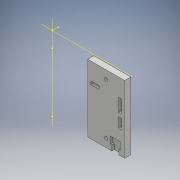
# Autodesk Inventor part: 1구버전
Saved by Autodesk Inventor 2018 (Build 220112000, 112)
## iProperties
Created: 2018-01-17
Part Number: 1구버전
Material: 일반
Document SubType Name: Modeling
Designer: NULL
Density: 1 g/cm^3
Appearance: 기본값
Author: NULL
Autodesk Inventor part; units mm, degrees
ref_plane "작업 평면1" through (0, 10, 0) normal (0, 1, 0) x (1, 0, 0)
sketch "스케치3" plane through (0, 10, 0) normal (0, 1, 0) x (1, 0, 0)
  line L0 (108.4435, 113.2704) -> (97.4435, 113.2704)
  line L1 (97.4435, 113.2704) -> (97.4435, 121.7204)
  line L2 (97.4435, 121.7204) -> (108.4435, 121.7204)
  line L3 (108.4435, 121.7204) -> (108.4435, 113.2704)
  line L4 (117.9435, 121.7204) -> (57.9435, 121.7204)
  line L5 (57.9435, 121.7204) -> (57.9435, 11.7204)
  line L6 (117.9435, 11.7204) -> (117.9435, 121.7204)
  line L7 (57.9435, 11.7204) -> (117.9435, 11.7204)
  line L8 (113.0685, 67.6907) -> (89.4185, 67.6907)
  line L9 (89.4185, 67.6907) -> (89.4185, 84.1907)
  line L10 (89.4185, 84.1907) -> (113.0685, 84.1907)
  line L11 (113.0685, 84.1907) -> (113.0685, 67.6907)
  line L12 (113.0684, 40.1407) -> (108.0685, 40.1407)
  line L13 (108.0685, 67.6907) -> (113.0685, 67.6907)
  line L14 (113.0684, 61.6907) -> (113.0684, 40.1407)
  line L15 (113.0685, 67.6907) -> (108.0685, 67.6907)
  line L16 (108.0685, 67.6907) -> (108.0685, 84.1907)
  line L17 (108.0685, 84.1907) -> (113.0685, 84.1907)
  line L18 (113.0685, 84.1907) -> (113.0685, 67.6907)
  line L19 (76.5185, 39.8907) -> (62.8185, 39.8907)
  line L20 (62.8185, 39.8907) -> (62.8185, 44.8907)
  line L21 (62.8185, 44.8907) -> (76.5185, 44.8907)
  line L22 (76.5185, 44.8907) -> (76.5185, 39.8907)
  line L23 (113.0684, 61.6907) -> (78.3675, 61.6907)
  circle A0 centre (87.9435, 25.2204) radius 2.6
  circle A1 centre (87.9435, 108.2204) radius 2.6
  line L24 (78.3675, 40.1407) -> (113.0684, 40.1407)
  line L25 (78.3675, 40.1407) -> (78.3675, 61.6907)
  line L26 (76.5185, 39.8907) -> (76.5185, 71.6407)
  line L27 (62.8185, 39.8907) -> (62.8185, 71.6407)
  line L28 (76.5185, 71.6407) -> (62.8185, 71.6407)
  line L29 (108.0685, 61.6907) -> (108.0685, 40.1407)
  point P0 (0, 0)
  dimension "d8" = 9.5
  dimension "d46" = 5.2
  dimension "d47" = 5.2
  constraints: 60 end point, 8 parallel, 6 horizontal, 4 perpendicular, 4 point on line, 2 centre point, 1 collinear, 1 vertical
  measures "d8" distance of L4.start L2.end
  measures "d46" diameter of A0
  measures "d47" diameter of A1
extrude "돌출2" add sketch "스케치3" against normal blind 10 contours L3 L4 L6 L7 L5 L1 L0 | L0 L1 L2 L3 | L8 L16 L10 L11 | L8 L9 L10 L16 | L12 L29 L23 L14 | L24 L25 L23 L29 | L19 L20 L21 L22 | L21 L27 L28 L26 | A0 | A1
sketch "스케치4" plane through (0, 10, 0) normal (0, 1, 0) x (1, 0, 0)
  point P0 (0, 0)
sketch "스케치5" plane through (117.9435, 10, -121.7204) normal (0, 0, -1) x (-1, 0, 0)
  point P0 (117.9435, -10)
extrude "돌출5" cut sketch "스케치3" against normal through all contours L0 L1 L2 L3
sketch "스케치6" plane through (0, 0, 0) normal (0, -1, 0) x (1, 0, 0)
  line L0 (57.9435, -121.7204) -> (97.4435, -121.7204) projected
  line L1 (97.4435, -121.7204) -> (57.9435, -121.7204) projected
  line L2 (113.0685, -71.6204) -> (108.0685, -71.6204) projected
  line L3 (113.0685, -80.2704) -> (113.0685, -71.6204) projected
  line L4 (78.3685, -80.2704) -> (113.0685, -80.2704) projected
  line L5 (78.3685, -58.4704) -> (78.3685, -80.2704) projected
  line L6 (113.0685, -58.4704) -> (78.3685, -58.4704) projected
  line L7 (113.0685, -67.1204) -> (113.0685, -58.4704) projected
  line L8 (108.0685, -67.1204) -> (113.0685, -67.1204) projected
  line L9 (108.0685, -71.6204) -> (108.0685, -67.1204) projected
  line L10 (117.9435, -121.7204) -> (108.4435, -121.7204) projected
  line L11 (111.4435, -108.7204) -> (94.443, -108.7204)
  line L12 (111.4435, -108.7204) -> (111.4435, -113.2704)
  line L13 (94.443, -108.7204) -> (94.443, -113.2704)
  line L14 (111.4435, -113.2704) -> (94.443, -113.2704)
  point P0 (0, 0)
  constraints: 8 end point, 2 vertical, 1 perpendicular
sketch "스케치7" plane through (0, 0, 0) normal (0, -1, 0) x (1, 0, 0)
  point P0 (0, 0)
sketch "스케치8" plane through (0, 0, 0) normal (0, -1, 0) x (1, 0, 0)
  point P0 (0, 0)
extrude "돌출6" cut sketch "스케치6" against normal blind 4 contours L12 L14 L13 L11
extrude "돌출7" add sketch "스케치3" against normal blind 6 contours L0 L1 L2 L3
sketch "스케치9" plane through (0, 0, 0) normal (0, -1, 0) x (1, 0, 0)
  line L0 (111.4435, -108.7204) -> (111.4435, -113.2704) projected
  line L1 (111.4435, -108.7204) -> (111.4435, -101.7204)
  line L2 (111.4435, -101.7204) -> (94.443, -101.7204)
  line L3 (94.443, -113.2704) -> (94.443, -108.7204) projected
  line L4 (94.443, -101.7204) -> (94.443, -108.7204)
  line L5 (94.443, -108.7204) -> (111.4435, -108.7204) projected
  line L6 (111.4435, -108.7204) -> (94.443, -108.7204)
  point P0 (0, 0)
  dimension "d25" = 7
  constraints: 8 end point, 2 perpendicular, 1 collinear, 1 vertical
  measures "d25" distance of L0.start L1.end
extrude "돌출8" cut sketch "스케치9" against normal blind 4
sketch "스케치10" plane through (0, 10, 0) normal (0, 1, 0) x (1, 0, 0)
  circle A0 centre (87.9435, 25.2204) radius 3.85
  circle A1 centre (87.9435, 108.2204) radius 3.85
  point P0 (0, 0)
  dimension "d28" = 7.7
  dimension "d29" = 7.7
  constraints: 2 centre point
  measures "d28" diameter of A0
  measures "d29" diameter of A1
ref_plane "작업 평면2" through (0, 10, 0) normal (0, 1, 0) x (1, 0, 0)
sketch "스케치12" plane through (0, 10, 0) normal (0, 1, 0) x (1, 0, 0)
  point P0 (0, 0)
ref_plane "작업 평면3" through (57.9435, 10, -25.2204) normal (0, 0, 1) x (1, 0, 0)
sketch "스케치13" plane through (57.9435, 10, -25.2204) normal (0, 0, 1) x (1, 0, 0)
  line L0 (30, 0) -> (30, -4)
  line L1 (30, 0) -> (33.65, 0)
  line L2 (33.65, 0) -> (30, -4)
  point P0 (-57.9435, -10)
  point P1 (32.25, 0)
  dimension "d35" = 4
  dimension "d36" = 3.65
  constraints: 6 end point, 1 vertical
  measures "d35" distance of L0.start L0.end
  measures "d36" distance of L0.start L1.end
sketch "스케치14" plane through (57.9435, 10, -25.2204) normal (0, 0, 1) x (1, 0, 0)
  point P0 (-57.9435, -10)
revolve "회전2" cut sketch "스케치13" angle 360 about axis through (87.9435, 10, -25.2204) along (0, -1, 0)
ref_plane "작업 평면4" through (57.9435, 10, -66.7204) normal (0, 0, 1) x (1, 0, 0)
mirror "미러1" about plane through (57.9435, 10, -66.7204) normal (0, 0, 1) of "회전2"
sketch "스케치15" plane through (0, 0, 0) normal (0, -1, 0) x (1, 0, 0)
  line L0 (108.6612, -121.7204) -> (97.1612, -121.7204)
  line L1 (97.1612, -121.7204) -> (97.1612, -113.2704)
  line L2 (108.6612, -121.7204) -> (108.6612, -113.2704)
  line L3 (97.1612, -113.2704) -> (108.6612, -113.2704)
  line L4 (97.4435, -113.2704) -> (94.443, -113.2704) projected
  point P0 (0, 0)
  constraints: 8 end point, 2 vertical, 1 collinear, 1 horizontal
extrude "돌출9" cut sketch "스케치15" against normal blind 4
extrude "돌출11" cut sketch "스케치3" against normal through all contours A0 | A1
extrude "돌출12" cut sketch "스케치3" against normal through all contours L8 L16 L10 L11 | L12 L29 L23 L14 | L19 L20 L21 L22
extrude "돌출13" cut sketch "스케치3" against normal blind 1.7 contours L8 L9 L10 L16 | L24 L25 L23 L29 | L21 L27 L28 L26
